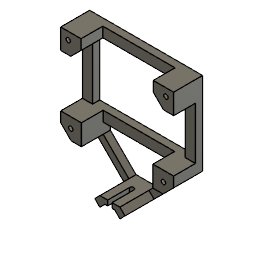
土台2(new) (Autodesk Fusion 360 design; units mm, degrees)
Autodesk Fusion 360 part; units mm, degrees
sketch "スケッチ1" plane through (0, 0, 0) normal (0, 0, 1) x (1, 0, 0)
  line L0 (-38.8909, 38.8909) -> (0, 0)
  line L1 (0, 0) -> (38.8909, 38.8909)
  line L2 (38.8909, 38.8909) -> (-38.8909, 38.8909) construction
  line L3 (0, 38.8909) -> (0, 0) construction
  line L4 (-24.5921, 31.6632) -> (-3.3789, 10.45)
  line L5 (-3.3789, 10.45) -> (3.3789, 10.45)
  line L6 (3.3789, 10.45) -> (24.5921, 31.6632)
  line L7 (24.5921, 31.6632) -> (24.5921, 38.8909)
  line L8 (-24.5921, 38.8909) -> (-24.5921, 31.6632)
  line L9 (-24.5921, 38.8909) -> (24.5921, 38.8909)
  line L10 (-38.8909, 38.8909) -> (-38.8909, 45.9909)
  line L11 (-31.8909, 45.9909) -> (31.8909, 45.9909)
  line L12 (38.8909, 45.9909) -> (38.8909, 38.8909)
  line L13 (31.8909, 45.9909) -> (-31.8909, 45.9909)
  line L14 (-38.8909, 45.9909) -> (-38.8909, 95.9909)
  line L15 (-38.8909, 95.9909) -> (38.8909, 95.9909)
  line L16 (38.8909, 95.9909) -> (38.8909, 45.9909)
  line L17 (38.8909, 45.9909) -> (-38.8909, 95.9909) construction
  line L18 (-38.8909, 45.9909) -> (38.8909, 95.9909) construction
  line L19 (-31.8909, 45.9909) -> (-31.8909, 81.9198)
  line L20 (-24.8198, 88.9909) -> (24.8198, 88.9909)
  line L21 (31.8909, 81.9198) -> (31.8909, 45.9909)
  line L22 (-24.8198, 88.9909) -> (-31.8909, 81.9198)
  line L23 (24.8198, 88.9909) -> (31.8909, 81.9198)
  point P0 (0, 70.9909)
  point P1 (0, 70.9909)
  dimension "d1" = 55
  dimension "d3" = 55
  dimension "d4" = 5
  dimension "d5" = 5
  dimension "d6" = 30
  dimension "d7" = 30
  dimension "d8" = 10.45
  dimension "d9" = 7.1
  dimension "d10" = 50
  dimension "d11" = 7
  dimension "d13" = 45
  dimension "d14" = 45
  dimension "d15" = 10
  dimension "d16" = 10
  dimension "d17" = 7
  dimension "d18" = 7
  dimension "d19" = 57.1
  dimension "d20" = 7.1
  constraint coincident L0.end L1.start
  constraint horizontal L2
  constraint midpoint L2 L3.start
  constraint perpendicular L3 L5
  constraint parallel L0 L4
  constraint parallel L1 L6
  constraint perpendicular L0 L1
  constraint vertical L8
  constraint vertical L7
  constraint coincident L2 L8.start
  constraint coincident L2 L7.end
  constraint coincident L0.start L2.end
  constraint horizontal L11
  constraint vertical L10
  constraint vertical L12
  constraint horizontal L13
  constraint perpendicular L13 L14
  constraint parallel L13 L15
  constraint parallel L14 L16
  constraint coincident L17 P1
  constraint coincident L18 P1
  constraint coincident L10.end L14.start
  constraint coincident P1 P0
  measures "d1" distance of L0.end L1.end
  measures "d3" distance of L0.start L0.end
  measures "d4" distance of L1 L6
  measures "d5" distance of L0 L4
  measures "d6" distance of L5.end L6.end
  measures "d7" distance of L4.start L4.end
  measures "d8" distance of L0.end L5
  measures "d9" distance of L9 L11
  measures "d10" distance of L12.start L15.end
  measures "d11" distance of L16 L21
  measures "d13" angle of L20 L22
  measures "d14" angle of L20 L23
  measures "d15" distance of L20.start L19.end
  measures "d16" distance of L20.end L21.start
  measures "d17" distance of L15 L20
  measures "d18" distance of L14 L19
  measures "d19" distance of L9 L15
  measures "d20" distance of L0.start L10.end
extrude "押し出し1" add sketch "スケッチ1" along normal mid plane 5
sketch "スケッチ2" plane through (0, 0, 2.5) normal (0, 0, 1) x (1, 0, 0)
  line L0 (-31.8909, 81.9198) -> (-24.8198, 88.9909)
  line L1 (-24.8198, 88.9909) -> (24.8198, 88.9909)
  line L2 (24.8198, 88.9909) -> (31.8909, 81.9198)
  line L3 (31.8909, 81.9198) -> (31.8909, 45.9909)
  line L4 (31.8909, 45.9909) -> (-31.8909, 45.9909)
  line L5 (-31.8909, 45.9909) -> (-31.8909, 81.9198)
  line L6 (-3.3789, 10.45) -> (-24.5921, 31.6632)
  line L7 (-24.5921, 31.6632) -> (-24.5921, 38.8909)
  line L8 (-24.5921, 38.8909) -> (24.5921, 38.8909)
  line L9 (24.5921, 38.8909) -> (24.5921, 31.6632)
  line L10 (24.5921, 31.6632) -> (3.3789, 10.45)
  line L11 (3.3789, 10.45) -> (-3.3789, 10.45)
  line L12 (-38.8909, 38.8909) -> (0, 0)
  line L13 (0, 0) -> (38.8909, 38.8909)
  line L14 (38.8909, 38.8909) -> (38.8909, 95.9909)
  line L15 (38.8909, 95.9909) -> (-38.8909, 95.9909)
  line L16 (-38.8909, 95.9909) -> (-38.8909, 38.8909)
  line L17 (-24.8198, 95.9909) -> (-24.8198, 88.9909)
  line L18 (-24.8198, 88.9909) -> (-31.8909, 81.9198)
  line L19 (-31.8909, 81.9198) -> (-38.8909, 81.9198)
  line L20 (-38.8909, 81.9198) -> (-38.8909, 95.9909)
  line L21 (-38.8909, 95.9909) -> (-24.8198, 95.9909)
  line L22 (24.8198, 95.9909) -> (24.8198, 88.9909)
  line L23 (24.8198, 88.9909) -> (31.8909, 81.9198)
  line L24 (31.8909, 81.9198) -> (38.8909, 81.9198)
  line L25 (38.8909, 81.9198) -> (38.8909, 95.9909)
  line L26 (38.8909, 95.9909) -> (24.8198, 95.9909)
  line L27 (-24.5921, 45.9909) -> (-24.5921, 31.6632)
  line L28 (-24.5921, 31.6632) -> (-31.6632, 31.6632)
  line L29 (-31.6632, 31.6632) -> (-38.8909, 38.8909)
  line L30 (-38.8909, 38.8909) -> (-38.8909, 45.9909)
  line L31 (-38.8909, 45.9909) -> (-24.5921, 45.9909)
  line L32 (24.5921, 45.9909) -> (24.5921, 31.6632)
  line L33 (24.5921, 31.6632) -> (31.6632, 31.6632)
  line L34 (31.6632, 31.6632) -> (38.8909, 38.8909)
  line L35 (38.8909, 38.8909) -> (38.8909, 45.9909)
  line L36 (38.8909, 45.9909) -> (24.5921, 45.9909)
  line L37 (-3.3789, 10.45) -> (-6.9145, 6.9145)
  line L38 (-6.9145, 6.9145) -> (0, 0)
  line L39 (0, 0) -> (6.9145, 6.9145)
  line L40 (6.9145, 6.9145) -> (3.3789, 10.45)
  line L41 (3.3789, 10.45) -> (-3.3789, 10.45)
  constraint coincident L15 L17.start
  constraint coincident L0.end L1.start
  constraint perpendicular L1 L17
  constraint coincident L0.start L5.end
  constraint coincident L16 L19.end
  constraint perpendicular L16 L19
  constraint coincident L15.end L16.start
  constraint coincident L15 L22.start
  constraint coincident L1.end L2.start
  constraint coincident L2.end L3.start
  constraint coincident L14 L24.end
  constraint perpendicular L14 L24
  constraint coincident L14.end L15.start
  constraint vertical L22
  constraint coincident L4 L27.start
  constraint coincident L6.end L7.start
  constraint coincident L12 L28.end
  constraint perpendicular L27 L28
  constraint vertical L27
  constraint coincident L16 L30.end
  constraint coincident L12.start L16.end
  constraint horizontal L31
  constraint vertical L32
  constraint perpendicular L32 L33
  constraint perpendicular L33 L35
  constraint coincident L4 L32.start
  constraint coincident L9.end L10.start
  constraint coincident L13 L33.end
  constraint coincident L14 L35.end
  constraint coincident L13.end L14.start
  constraint horizontal L36
  constraint coincident L6.start L11.end
  constraint coincident L12 L37.end
  constraint perpendicular L12 L37
  constraint perpendicular L12 L39
  constraint coincident L10.end L11.start
  constraint coincident L13 L39.end
  constraint coincident L12.end L13.start
  constraint perpendicular L13 L40
extrude "押し出し2" add sketch "スケッチ2" along normal blind 15 contours L0 L15 L16 L17 L18 L19 L20 L21 | L4 L7 L12 L16 L27 L28 L29 L30 L31 | L2 L14 L15 L22 L23 L24 L25 L26 | L4 L9 L13 L14 L32 L33 L34 L35 L36
extrude "押し出し3" add sketch "スケッチ2" along normal blind 60 contours L11 L12 L13 L37 L38 L39 L40 L41
sketch "スケッチ3" plane through (0, 0, -2.5) normal (0, 0, -1) x (-1, 0, 0)
  line L0 (24.8198, 88.9909) -> (31.8909, 81.9198)
  line L1 (31.8909, 81.9198) -> (31.8909, 45.9909)
  line L2 (31.8909, 45.9909) -> (-31.8909, 45.9909)
  line L3 (-31.8909, 45.9909) -> (-31.8909, 81.9198)
  line L4 (-31.8909, 81.9198) -> (-24.8198, 88.9909)
  line L5 (-24.8198, 88.9909) -> (24.8198, 88.9909)
  line L6 (24.5921, 31.6632) -> (3.3789, 10.45)
  line L7 (3.3789, 10.45) -> (-3.3789, 10.45)
  line L8 (-3.3789, 10.45) -> (-24.5921, 31.6632)
  line L9 (-24.5921, 31.6632) -> (-24.5921, 38.8909)
  line L10 (-24.5921, 38.8909) -> (24.5921, 38.8909)
  line L11 (24.5921, 38.8909) -> (24.5921, 31.6632)
  line L12 (0, 0) -> (38.8909, 38.8909)
  line L13 (38.8909, 38.8909) -> (38.8909, 95.9909)
  line L14 (38.8909, 95.9909) -> (-38.8909, 95.9909)
  line L15 (-38.8909, 95.9909) -> (-38.8909, 38.8909)
  line L16 (-38.8909, 38.8909) -> (0, 0)
  line L17 (-38.8909, 95.9909) -> (-28.3553, 85.4553) construction
  line L18 (38.8909, 95.9909) -> (28.3553, 85.4553) construction
  circle A0 centre (-33.6231, 90.7231) radius 3.5
  circle A1 centre (33.6231, 90.7231) radius 3.5
  circle A2 centre (-31.8909, 38.8909) radius 3.5
  circle A3 centre (31.8909, 38.8909) radius 3.5
  line L19 (-24.5921, 38.8909) -> (-38.8909, 38.8909) construction
  line L20 (-31.8909, 45.9909) -> (-31.8909, 31.8909) construction
  line L21 (24.5921, 38.8909) -> (38.8909, 38.8909) construction
  line L22 (31.8909, 45.9909) -> (31.8909, 31.8909) construction
  circle A4 centre (-31.8909, 38.8909) radius 1.5
  circle A5 centre (31.8909, 38.8909) radius 1.5
  circle A6 centre (33.6231, 90.7231) radius 1.5
  circle A7 centre (-33.6231, 90.7231) radius 1.5
  dimension "d27" = 7
  dimension "d28" = 7
  dimension "d29" = 7
  dimension "d30" = 7
  dimension "d31" = 3
  dimension "d32" = 3
  dimension "d33" = 3
  dimension "d34" = 3
  constraint coincident L14.end L15.start
  constraint midpoint L4 L17.end
  constraint coincident L13.end L14.start
  constraint midpoint L0 L18.end
  constraint midpoint L17 A0.centre
  constraint midpoint L18 A1.centre
  constraint coincident L9.end L10.start
  constraint coincident L15.end L16.start
  constraint coincident L2.end L3.start
  constraint coincident L16 L20.end
  constraint perpendicular L19 L20
  constraint coincident A2.centre L19
  constraint coincident A2.centre L20
  constraint coincident L10.end L11.start
  constraint coincident L12.end L13.start
  constraint coincident L1.end L2.start
  constraint coincident L12 L22.end
  constraint perpendicular L21 L22
  constraint coincident A3.centre L22
  constraint coincident A3.centre L21
  constraint concentric A2 A4
  constraint concentric A3 A5
  constraint concentric A1 A6
  constraint concentric A0 A7
  measures "d27" diameter of A0
  measures "d28" diameter of A1
  measures "d29" diameter of A2
  measures "d30" diameter of A3
  measures "d31" diameter of A4
  measures "d32" diameter of A5
  measures "d33" diameter of A6
  measures "d34" diameter of A7
extrude "押し出し4" cut sketch "スケッチ3" against normal blind 25 contours A4 | A5 | A6 | A7
extrude "押し出し7" cut 1 faces at (0, 6.9667, 62.5) along direction (0, 0, -1) blind 65
sketch "スケッチ8" plane through (0, 0, 2.5) normal (0, 0, 1) x (1, 0, 0)
  line L0 (-6.9145, 6.9145) -> (-3.3789, 10.45)
  line L1 (-3.3789, 10.45) -> (-24.5921, 31.6632)
  line L2 (-24.5921, 31.6632) -> (-31.6632, 31.6632)
  line L3 (-31.6632, 31.6632) -> (-6.9145, 6.9145)
  line L4 (3.3789, 10.45) -> (6.9145, 6.9145)
  line L5 (24.5921, 31.6632) -> (3.3789, 10.45)
  line L6 (6.9145, 6.9145) -> (31.6632, 31.6632)
  line L7 (-3.3789, 10.45) -> (3.3789, 10.45)
  line L8 (-6.9145, 13.9855) -> (6.9145, 13.9855)
  line L9 (6.9145, 13.9855) -> (10.45, 10.45)
  line L10 (-6.9145, 13.9855) -> (-10.45, 10.45)
  dimension "d52" = 5
  dimension "d53" = 5
  constraint coincident L0.end L1.start
  constraint coincident L4.start L5.end
  constraint coincident L1 L8.start
  constraint coincident L5 L8.end
  constraint coincident L6 L9.end
  constraint coincident L3 L10.end
  constraint perpendicular L1 L10
  constraint perpendicular L6 L9
  measures "d52" distance of L0 L10
  measures "d53" distance of L4 L9
extrude "押し出し9" add sketch "スケッチ8" against normal blind 5 contours L1 L5 L7 L8
extrude "押し出し10" add sketch "スケッチ8" along normal blind 20 contours L0 L1 L3 L10 | L1 L5 L7 L8 | L4 L5 L6 L9
sketch "スケッチ9" plane through (0, 10.45, 0) normal (0, -1, 0) x (1, 0, 0)
  line L0 (-3.3789, 22.5) -> (-3.3789, -2.5)
  line L1 (-3.3789, -2.5) -> (3.3789, -2.5)
  line L2 (3.3789, -2.5) -> (3.3789, 22.5)
  line L3 (3.3789, 22.5) -> (-3.3789, 22.5)
  arc A0 (-1.5, 7.5) -> (1.5, 7.5) centre (0, 7.5) ccw
  line L4 (0, 7.5) -> (0, -2.5) construction
  line L5 (-1.5, 7.5) -> (-1.5, 22.5)
  line L6 (1.5, 22.5) -> (1.5, 7.5)
  dimension "d58" = 10
  dimension "d59" = 1.5
  constraint coincident A0.centre L4.start
  constraint midpoint L1 L4.end
  constraint vertical L4
  constraint coincident L3 L5.end
  constraint tangent A0 L5
  constraint coincident L3 L6.start
  constraint tangent A0 L6
  constraint vertical L6
  constraint vertical L5
  measures "d58" distance of A0.centre L4.end
  measures "d59" radius of A0
extrude "押し出し11" cut sketch "スケッチ9" against normal blind 4 contours L3 A0 L5 L6
extrude "押し出し12" add sketch "スケッチ3" against normal blind 4 contours A4 | A5 | A6 | A7
